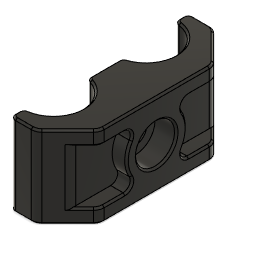
Apollo Yoke Lock P3 [(P)MPLA000000158] v2 (Autodesk Fusion 360 design; units mm, degrees)
Autodesk Fusion 360 part; units mm, degrees
sketch "Sketch1" plane through (0, 0, 0) normal (0, 1, 0) x (1, 0, 0)
  circle A0 centre (0, -13) radius 8
  circle A1 centre (0, 13) radius 8
  line L0 (3, 5.841) -> (3, -5.7657)
  line L1 (-1.1294, 25) -> (-1.1294, -25)
  line L2 (12, 20) -> (12, -20)
  line L3 (-1.1294, -25) -> (7, -25)
  circle A2 centre (0, 13) radius 8.2
  circle A3 centre (0, -13) radius 8.2
  line L4 (-1.1294, 25) -> (7, 25)
  line L5 (-8.1131, 21.2) -> (3.4058, 21.2)
  line L6 (-8.2208, -21.2) -> (2.5446, -21.2)
  line L7 (7, 25) -> (12, 20)
  line L8 (7, -25) -> (12, -20)
  line L9 (-0.1294, -25) -> (-0.1294, 25)
  line L10 (1.5, -6.0793) -> (1.5, 6.3575)
  point P0 (12, 25)
  point P1 (12, -25)
  dimension "d63" = 16
  dimension "d64" = 16
  dimension "d65" = 26
  dimension "d4" = 13
  dimension "d5" = 0.2
  dimension "d6" = 0.2
  dimension "d7" = 50
  dimension "d8" = 25
  dimension "d22" = 13.1294
  dimension "d23" = 3
  dimension "d24" = 9
  dimension "d25" = 5
  dimension "d26" = 5
  dimension "d27" = 5
  dimension "d28" = 5
  dimension "d51" = 1
  dimension "d53" = 1.5
  constraint vertical A0.centre A1.centre
  constraint vertical origin A1.centre
  constraint vertical L0
  constraint vertical L1
  constraint vertical L2
  constraint horizontal L3
  constraint horizontal L4
  constraint horizontal L5
  constraint horizontal L6
  constraint tangent A2 L5
  constraint tangent A3 L6
  constraint coincident P0 L4
  constraint coincident P0 L2
  constraint coincident L3 P1
  constraint coincident L2 P1
  constraint coincident L3 L9.start
  constraint coincident L4 L9.end
  constraint perpendicular L4 L9
  constraint vertical L10
  measures "d63" diameter of A1
  measures "d64" diameter of A0
  measures "d65" distance of A0.centre A1.centre
  measures "d4" vertical distance of origin A1.centre
  measures "d7" distance of L3 L4
  measures "d8" distance of origin L3
  measures "d22" distance of L1 L2
  measures "d23" distance of origin L0
  measures "d24" distance of L0 L2
  measures "d25" distance of P0 L4.end
  measures "d26" distance of P0 L2.start L5
  measures "d27" distance of P1 L3.end
  measures "d28" distance of P1 L2.end
  measures "d51" distance of L1 L9
  measures "d53" distance of L0 L10
extrude "Extrude1" add sketch "Sketch1" along normal blind 23 contours L0 A2 A3 L10 | L0 L2 L3 A2 A3 L4 L5 L6 L7 L8 L9 | A3 L6 L9 | A2 L5 L9
fillet "Fillet1" radius 3 4 edges at (7, 11.5, -25) (12, 11.5, -20) (12, 11.5, 20) (7, 11.5, 25)
fillet "Fillet2" radius 1.5 6 edges at (-0.1294, 11.5, 21.199) (-0.1294, 11.5, 25) (-0.1294, 11.5, -21.199) (-0.1294, 11.5, -25) (1.5, 11.5, 4.9384) (1.5, 11.5, -4.9384)
sketch "Sketch2" plane through (12, 0, 0) normal (1, 0, 0) x (0, 0, -1)
  line L0 (-18.7574, 0) -> (18.7574, 0)
  line L1 (18.7574, 23) -> (-18.7574, 23)
  circle A0 centre (0, 11.5) radius 3.2
  circle A1 centre (0, 11.5) radius 5.5
  line L2 (-18.7574, 23) -> (-18.7574, 0)
  line L3 (18.7574, 0) -> (18.7574, 23)
  line L4 (-18.7574, 11.5) -> (18.7574, 11.5)
  dimension "d15" = 6.4
  dimension "d17" = 11
  constraint vertical origin A0.centre
  constraint concentric A0 A1
  constraint midpoint L2 L4.start
  constraint midpoint L3 L4.end
  constraint midpoint A0.centre L4
  measures "d15" diameter of A0
  measures "d17" diameter of A1
extrude "Extrude2" cut sketch "Sketch2" against normal blind 13 contours A0 L4 | A0 L4
extrude "Extrude3" cut sketch "Sketch2" against normal blind 2 contours A0 A1 L4 | A0 A1 L4
sketch "Sketch6" plane through (0, 0, 0) normal (0, -1, 0) x (1, 0, 0)
  arc A0 (1.5, -3.7756) -> (2.5361, -5.202) centre (3, -3.7756) ccw
  arc A1 (1.1586, -21.1177) -> (2.5361, -5.202) centre (0, -13) ccw
  arc A2 (1.1586, -21.1177) -> (-0.1294, -22.6027) centre (1.3706, -22.6027) ccw
  line L0 (-0.1294, -22.6027) -> (-0.1294, -23.5)
  arc A3 (-0.1294, -23.5) -> (1.3706, -25) centre (1.3706, -23.5) ccw
  line L1 (1.3706, -25) -> (5.7574, -25)
  arc A4 (5.7574, -25) -> (7.8787, -24.1213) centre (5.7574, -22) ccw
  line L2 (7.8787, -24.1213) -> (11.1213, -20.8787)
  arc A5 (11.1213, -20.8787) -> (12, -18.7574) centre (9, -18.7574) ccw
  line L3 (12, -18.7574) -> (12, 18.7574)
  arc A6 (12, 18.7574) -> (11.1213, 20.8787) centre (9, 18.7574) ccw
  line L4 (11.1213, 20.8787) -> (7.8787, 24.1213)
  arc A7 (7.8787, 24.1213) -> (5.7574, 25) centre (5.7574, 22) ccw
  line L5 (5.7574, 25) -> (1.3706, 25)
  arc A8 (1.3706, 25) -> (-0.1294, 23.5) centre (1.3706, 23.5) ccw
  line L6 (-0.1294, 23.5) -> (-0.1294, 22.6027)
  arc A9 (-0.1294, 22.6027) -> (1.1586, 21.1177) centre (1.3706, 22.6027) ccw
  arc A10 (2.5361, 5.202) -> (1.1586, 21.1177) centre (0, 13) ccw
  arc A11 (2.5361, 5.202) -> (1.5, 3.7756) centre (3, 3.7756) ccw
  line L7 (1.5, 3.7756) -> (1.5, -3.7756)
  line L8 (10.1153, 21.8847) -> (15.1213, 16.8787)
  line L9 (16, 14.7574) -> (16, -14.7574)
  line L10 (15.1213, -16.8787) -> (9.5, -22.5)
  arc A12 (16, 14.7574) -> (15.1213, 16.8787) centre (13, 14.7574) ccw
  arc A13 (15.1213, -16.8787) -> (16, -14.7574) centre (13, -14.7574) ccw
  dimension "d54" = 4
  dimension "d55" = 3
  constraint coincident L4 L8.start
  constraint parallel L3 L9
  constraint midpoint L2 L10.end
  constraint collinear L2 L10
  constraint collinear L4 L8
  constraint tangent L8 A12
  constraint tangent L9 A12
  constraint tangent L9 A13
  constraint tangent L10 A13
  constraint equal A12 A13
  measures "d54" distance of L3 L9
  measures "d55" radius of A12
extrude "Extrude6" add sketch "Sketch6" against normal blind 4 contours A5 L3 A6 L8 L9 L10 A12 A13
extrude "Extrude7" add sketch "Sketch6" along normal blind 4 from surface at -23 contours A5 L3 A6 L8 L9 L10 A12 A13
sketch "Sketch7" plane through (12, 0, 0) normal (1, 0, 0) x (0, 0, -1)
  circle A0 centre (0, 11.5) radius 5.5
  line L0 (18.7574, 19) -> (-18.7574, 19)
  line L1 (-18.7574, 19) -> (-18.7574, 4)
  line L2 (-18.7574, 4) -> (18.7574, 4)
  line L3 (18.7574, 4) -> (18.7574, 19)
  circle A1 centre (0, 11.5) radius 8.5
  dimension "d61" = 3
extrude "Extrude8" add sketch "Sketch7" along normal up to surface (4 mm away) contours L0 L2 A1
fillet "Fillet4" radius 2 4 edges at (14, 19, 4) (14, 4, 4) (14, 19, -4) (14, 4, -4)
chamfer "Chamfer5" distance 0.5 angle 45 59 edges at (8.1695, 0, 13.707) (1.7864, 0, 4.6571) (1.5, 0, 0) (1.7864, 0, -4.6571) (8.1695, 0, -13.707) (0.2374, 0, -21.6198) (-0.1294, 0, -23.0513) (0.3099, 0, -24.5607) (3.564, 0, -25) (6.9054, 0, -24.7716) (11.5, 0, -20.5) (15.7716, 0, -15.9054) (16, 0, 0) (15.7716, 0, 15.9054) (11.5, 0, 20.5) (6.9054, 0, 24.7716) (3.564, 0, 25) (0.3099, 0, 24.5607) (-0.1294, 0, 23.0513) (0.2374, 0, 21.6198) (8.1695, 23, 13.707) (0.2374, 23, 21.6198) (-0.1294, 23, 23.0513) (0.3099, 23, 24.5607) (3.564, 23, 25) (6.9054, 23, 24.7716) (11.5, 23, 20.5) (15.7716, 23, 15.9054) (16, 23, 0) (15.7716, 23, -15.9054) (11.5, 23, -20.5) (6.9054, 23, -24.7716) (3.564, 23, -25) (0.3099, 23, -24.5607) (-0.1294, 23, -23.0513) (0.2374, 23, -21.6198) (8.1695, 23, -13.707) (1.7864, 23, -4.6571) (1.5, 23, 0) (1.7864, 23, 4.6571) (16, 19, 11.8508) (15.7716, 19, 15.9054) (13.1213, 19, 18.8787) (13.1213, 4, 18.8787) (15.7716, 4, 15.9054) (16, 4, 11.8508) (16, 5.0241, 7.1985) (16, 11.5, 8.5) (16, 17.9759, 7.1985) (16, 19, -11.8508) (16, 17.9759, -7.1985) (16, 11.5, -8.5) (16, 5.0241, -7.1985) (16, 4, -11.8508) (15.7716, 4, -15.9054) (13.1213, 4, -18.8787) (13.1213, 19, -18.8787) (15.7716, 19, -15.9054) (16, 9.5111, 5.1278)
equation "d4 = d65 / 2"
equation "d8 = d7 / 2"
equation "d26 = d25"
equation "d28 = d27"
